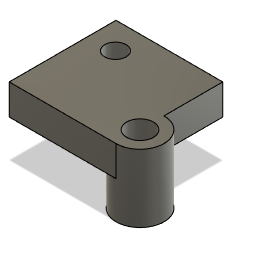
Screenmount (Autodesk Fusion 360 design; units mm, degrees)
Autodesk Fusion 360 part; units mm, degrees
sketch "Sketch1" plane through (0, 0, 0) normal (0, 1, 0) x (1, 0, 0)
  circle A0 centre (0, 0) radius 3
  circle A1 centre (0, 0) radius 1.15
  circle A2 centre (0, 0) radius 4.5
  dimension "d1" = 6
  dimension "d2" = 2.3
  dimension "d3" = 9
  constraint coincident A0.centre A1.centre
  constraint concentric A0 A1
  constraint concentric A0 A2
  measures "d1" diameter of A0
  measures "d2" diameter of A1
  measures "d3" diameter of A2
extrude "Extrude1" add sketch "Sketch1" along normal blind 7 contours A2
sketch "Sketch2" plane through (0, 7, 0) normal (0, 1, 0) x (-1, 0, 0)
  circle A0 centre (0, 0) radius 3
  circle A1 centre (0, 0) radius 4.5
  circle A2 centre (0, 0) radius 2.75
  circle A3 centre (0, 0) radius 1.25
  dimension "d6" = 2.5
  constraint coincident A0.centre A1.centre
  constraint concentric A2 A3
  measures "d6" diameter of A3
extrude "Extrude2" add sketch "Sketch2" against normal blind 2.9 contours A0 | A2
sketch "Sketch3" plane through (0, 7, 0) normal (0, 1, 0) x (-1, 0, 0)
  circle A0 centre (0, 0) radius 1.25
  circle A1 centre (0, 0) radius 4.5
  line L0 (0, 4.5) -> (20, 4.5)
  line L1 (20, 4.5) -> (20, -15.5)
  line L2 (20, -15.5) -> (0, -15.5)
  line L3 (0, -15.5) -> (0, -4.5)
  dimension "d9" = 20
  dimension "d10" = 20
  constraint coincident A1 L0.start
  constraint horizontal L0
  constraint perpendicular L0 L1
  constraint perpendicular L1 L2
  constraint coincident A1 L3.end
  constraint perpendicular L2 L3
  measures "d9" distance of L0.start L0.end
  measures "d10" distance of L0.end L1.end
extrude "Extrude3" add sketch "Sketch3" along normal blind 3
sketch "Sketch4" plane through (0, 10, 0) normal (0, 1, 0) x (-1, 0, 0)
  circle A0 centre (0, 0) radius 1.25
  arc A1 (0, 4.5) -> (0, -4.5) centre (0, 0) ccw
  line L0 (0, -4.5) -> (0, -15.5)
  line L1 (0, -15.5) -> (20, -15.5)
  line L2 (20, -15.5) -> (20, 4.5)
  line L3 (20, 4.5) -> (0, 4.5)
  circle A2 centre (0, 0) radius 2.5
  dimension "d13" = 5
  constraint concentric A0 A2
  measures "d13" diameter of A2
extrude "Extrude4" cut sketch "Sketch4" against normal blind 2 contours A2
sketch "Sketch5" plane through (0, 10, 0) normal (0, 1, 0) x (-1, 0, 0)
  circle A0 centre (0, 0) radius 2.5
  arc A1 (0, 4.5) -> (0, -4.5) centre (0, 0) ccw
  line L0 (0, -4.5) -> (0, -15.5)
  line L1 (0, -15.5) -> (20, -15.5)
  line L2 (20, -15.5) -> (20, 4.5)
  line L3 (20, 4.5) -> (0, 4.5)
  line L4 (0, 0) -> (15.1, 0)
  line L5 (15.1, 0) -> (15.1, -8.5)
  line L6 (15.1, -8.5) -> (15.1, -10.5)
  circle A2 centre (15.1, -10.5) radius 2
  dimension "d16" = 15.1
  dimension "d17" = 8.5
  dimension "d18" = 90
  dimension "d19" = 2
  dimension "d20" = 4
  constraint coincident A0.centre A1.centre
  constraint horizontal L4
  constraint parallel L5 L6
  constraint coincident L6.end A2.centre
  measures "d16" distance of A0.centre L4.end
  measures "d17" distance of L4.end L5.end
  measures "d18" angle of L4 L5
  measures "d19" distance of L5.end L6.end
  measures "d20" diameter of A2
extrude "Extrude5" add sketch "Sketch5" along normal blind 2.7
extrude "Extrude6" cut 1 faces at (-14.7065, 10, -9.6829) along direction (0, -1, 0) blind 2
sketch "Sketch6" plane through (0, 8, 0) normal (0, 1, 0) x (-1, 0, 0)
  circle A0 centre (15.1, -10.5) radius 2
  circle A1 centre (15.1, -10.5) radius 1.6
  dimension "d25" = 3.2
  constraint concentric A0 A1
  measures "d25" diameter of A1
extrude "Extrude7" cut sketch "Sketch6" against normal blind 14 contours A1
extrude "Extrude8" cut 1 faces at (-2.0694, 8, -0.1863) along direction (0, -1, 0) blind 2
equation "d7 = -( 7 mm - 4.1 mm )"
equation "d16 = 13.5 mm + 1.6 mm"
equation "d21 = 5.7 mm - 3 mm"
